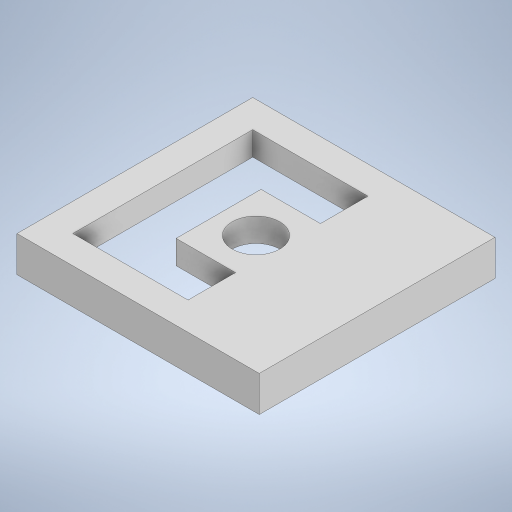
# Autodesk Inventor part: cam_socket
Saved by Autodesk Inventor 2024.3 (Build 283343000, 343)
## iProperties
Created: 2024-08-03
Part Number: cam_socket
Material: Generic
Document SubType Name: Modeling
Designer: compu
Density: 1 g/cm^3
Appearance: Default
Author: compu
Autodesk Inventor part; units mm, degrees
ref_plane "YZ Plane" through (0, 0, 0) normal (1, 0, 0) x (0, 1, 0)
ref_plane "XZ Plane" through (0, 0, 0) normal (0, 1, 0) x (-1, 0, 0)
ref_plane "XY Plane" through (0, 0, 0) normal (0, 0, 1) x (1, 0, 0)
sketch "Sketch1" plane through (0, 0, 0) normal (0, 1, 0) x (-1, 0, 0)
  line L0 (17.7, -17.15) -> (-17.7, -17.15)
  line L1 (-17.7, -17.15) -> (-17.7, 17.15)
  line L2 (-17.7, 17.15) -> (17.7, 17.15)
  line L3 (17.7, 17.15) -> (17.7, -17.15)
  line L4 (28.56, 0) -> (-28.56, 0) projected
  line L5 (0, -27.79) -> (0, 27.79) projected
  line L6 (-3.7, 7.15) -> (6.3, 7.15)
  line L7 (6.3, 7.15) -> (6.3, -7.15)
  line L8 (6.3, -7.15) -> (-3.7, -7.15)
  line L9 (-3.7, -15.15) -> (-3.7, -7.15)
  line L10 (-3.7, 7.15) -> (-3.7, 15.15)
  line L11 (15.7, 15.15) -> (-3.7, 15.15)
  line L12 (-3.7, -15.15) -> (15.7, -15.15)
  line L13 (15.7, -15.15) -> (15.7, 15.15)
  line L14 (-18.4, -17.85) -> (18.4, -17.85)
  line L15 (18.4, -17.85) -> (18.4, 17.85)
  line L16 (18.4, 17.85) -> (-18.4, 17.85)
  line L17 (-18.4, 17.85) -> (-18.4, -17.85)
  line L18 (20.4, -19.85) -> (-20.4, -19.85)
  line L19 (-20.4, -19.85) -> (-20.4, 19.85)
  line L20 (-20.4, 19.85) -> (20.4, 19.85)
  line L21 (20.4, 19.85) -> (20.4, -19.85)
  point P0 (0, 0)
  dimension "d0" = 34.3
  dimension "d1" = 35.4
  dimension "d3" = 10
  dimension "d4" = 10
  dimension "d5" = 24
  dimension "d6" = 14
  dimension "d7" = 14
  dimension "d8" = 2
  dimension "d9" = 2
  dimension "d10" = 2
  dimension "d11" = 0.7
  dimension "d12" = 2
  constraints: 40 end point, 11 perpendicular, 6 parallel, 2 horizontal, 8 other
  measures "d0" distance of L2.end L0.start
  measures "d1" distance of L0.start L0.end
  measures "d3" distance between parallel lines of L2 L6
  measures "d4" distance between parallel lines of L0 L8
  measures "d5" distance between parallel lines of L1 L7
  measures "d6" distance between parallel lines of L1 L9
  measures "d7" distance between parallel lines of L1 L10
  measures "d8" distance between parallel lines of L2 L11
  measures "d9" distance between parallel lines of L0 L12
  measures "d10" distance between parallel lines of L3 L13
  measures "d11" distance between parallel lines of L0 L14
  measures "d12" distance between parallel lines of L14 L18
extrude "Extrusion1" add sketch "Sketch1" along normal blind 4 contours L3 L4 L15 L14 L5 L0 | L0 L5 L12 L13 L4 L3 | L5 L14 L17 L4 L1 L0 | L0 L1 L4 L5 L8 L9 L12 | L4 L13 L11 L5 L2 L3 | L3 L2 L5 L16 L15 L4 | L14 L15 L4 L21 L18 L5 | L5 L18 L19 L4 L17 L14 | L15 L16 L5 L20 L21 L4 | L4 L17 L16 L5 L2 L1 | L1 L2 L5 L11 L10 L6 L4 | L5 L4 L7 L8 | L4 L5 L6 L7 | L4 L19 L20 L5 L16 L17
extrude "Extrusion2" add sketch "Sketch1" against normal blind 2 contours L14 L15 L4 L21 L18 L5 | L5 L18 L19 L4 L17 L14 | L15 L16 L5 L20 L21 L4 | L4 L19 L20 L5 L16 L17
sketch "Sketch3" plane through (0, 4, 0) normal (0, 1, 0) x (1, 0, 0)
  line L0 (-28.56, 0) -> (28.56, 0) projected
  line L1 (0, 27.79) -> (0, -27.79) projected
  circle A0 centre (0, 0) radius 4
  dimension "d17" = 8
  constraints: 1 centre point, 1 coincident
  measures "d17" diameter of A0
extrude "Extrusion3" cut sketch "Sketch3" against normal blind 4
body "Solid1"
